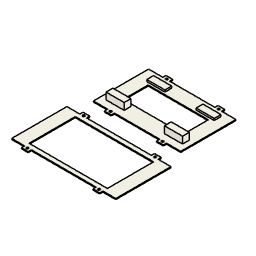
SD XL Bracket (Autodesk Fusion 360 design; units mm, degrees)
Autodesk Fusion 360 part; units mm, degrees
note: some values were not read from the file. Set by a fixed rule: which sketch regions a step uses.
sketch "Sketch1" plane through (0, 0, 0) normal (0, 0, 1) x (1, 0, 0) in component "SD XL Back"
  line L0 (0, 0) -> (0, 5) construction
  line L1 (-91.5, 117) -> (91.5, 117)
  line L2 (91.5, 117) -> (91.5, 5)
  line L3 (91.5, 5) -> (-91.5, 5)
  line L4 (-91.5, 5) -> (-91.5, 117)
  line L5 (-74.5, 111) -> (-34.5, 111)
  line L6 (-34.5, 111) -> (-34.5, 96)
  line L7 (-34.5, 96) -> (-74.5, 96)
  line L8 (-74.5, 96) -> (-74.5, 111)
  line L9 (34.5, 111) -> (74.5, 111)
  line L10 (74.5, 111) -> (74.5, 96)
  line L11 (74.5, 96) -> (34.5, 96)
  line L12 (34.5, 96) -> (34.5, 111)
  line L13 (-84.5, 31) -> (-44.5, 31)
  line L14 (-44.5, 31) -> (-44.5, 16)
  line L15 (-44.5, 16) -> (-84.5, 16)
  line L16 (-84.5, 16) -> (-84.5, 31)
  line L17 (44.5, 31) -> (84.5, 31)
  line L18 (84.5, 31) -> (84.5, 16)
  line L19 (84.5, 16) -> (44.5, 16)
  line L20 (44.5, 16) -> (44.5, 31)
  line L21 (-66.5, 91) -> (66.5, 91)
  line L22 (66.5, 91) -> (66.5, 36)
  line L23 (66.5, 36) -> (-66.5, 36)
  line L24 (-66.5, 36) -> (-66.5, 91)
  line L25 (0, 117) -> (0, 91) construction
  line L26 (0, 5) -> (0, 36) construction
  line L27 (-96.5, 0) -> (-96.5, 122)
  line L28 (96.5, 122) -> (96.5, 0)
  line L29 (-65, 117) -> (-50, 117)
  line L30 (-50, 117) -> (-50, 129)
  line L31 (-50, 129) -> (-65, 129)
  line L32 (-65, 129) -> (-65, 117)
  line L33 (50, 117) -> (65, 117)
  line L34 (65, 117) -> (65, 129)
  line L35 (65, 129) -> (50, 129)
  line L36 (50, 129) -> (50, 117)
  line L37 (57.5, 129) -> (57.5, 117) construction
  line L38 (-57.5, 129) -> (-57.5, 117) construction
  circle A0 centre (57.5, 123) radius 2.5
  circle A1 centre (-57.5, 123) radius 2.5
  line L39 (-96.5, 122) -> (-65, 122)
  line L40 (-50, 122) -> (50, 122)
  line L41 (65, 122) -> (96.5, 122)
  line L42 (-50, 5) -> (-65, 5)
  line L43 (-65, 5) -> (-65, -7)
  line L44 (-65, -7) -> (-50, -7)
  line L45 (-50, -7) -> (-50, 5)
  line L46 (50, 5) -> (65, 5)
  line L47 (65, 5) -> (65, -7)
  line L48 (65, -7) -> (50, -7)
  line L49 (50, -7) -> (50, 5)
  line L50 (-57.5, 5) -> (-57.5, -7) construction
  line L51 (57.5, 5) -> (57.5, -7) construction
  circle A2 centre (-57.5, -1) radius 2.5
  circle A3 centre (57.5, -1) radius 2.5
  line L52 (-65, 0) -> (-96.5, 0)
  line L53 (96.5, 0) -> (65, 0)
  line L54 (50, 0) -> (-50, 0)
  dimension "d1" = 5
  dimension "d2" = 183
  dimension "d5" = 112
  dimension "d8" = 40
  dimension "d9" = 15
  dimension "d10" = 17
  dimension "d11" = 17
  dimension "d12" = 7
  dimension "d13" = 7
  dimension "d14" = 11
  dimension "d15" = 11
  dimension "d19" = 25
  dimension "d28" = 12
  dimension "d29" = 15
  dimension "d31" = 50
  dimension "d32" = 50
  dimension "d33" = 5
  dimension "d41" = 6
  dimension "d42" = 5
  dimension "d43" = 5
  dimension "d44" = 26
  constraint coincident L0.start origin
  constraint vertical L0
  constraint horizontal L1
  constraint vertical L2
  constraint horizontal L3
  constraint vertical L4
  constraint midpoint L0.end L3
  constraint horizontal L5
  constraint vertical L6
  constraint horizontal L7
  constraint vertical L8
  constraint horizontal L9
  constraint vertical L10
  constraint horizontal L11
  constraint vertical L12
  constraint equal L7 L11
  constraint equal L6 L12
  constraint horizontal L13
  constraint vertical L14
  constraint horizontal L15
  constraint vertical L16
  constraint horizontal L17
  constraint vertical L18
  constraint horizontal L19
  constraint vertical L20
  constraint equal L7 L15
  constraint equal L7 L19
  constraint equal L6 L14
  constraint equal L6 L18
  constraint horizontal L21
  constraint vertical L22
  constraint horizontal L23
  constraint vertical L24
  constraint midpoint L1 L25.start
  constraint perpendicular L1 L25
  constraint midpoint L21 L25.end
  constraint perpendicular L3 L26
  constraint midpoint L23 L26.end
  constraint horizontal L29
  constraint vertical L30
  constraint horizontal L31
  constraint vertical L32
  constraint coincident L1 L29.start
  constraint horizontal L33
  constraint vertical L34
  constraint horizontal L35
  constraint vertical L36
  constraint coincident L1 L33.start
  constraint equal L30 L36
  constraint equal L31 L35
  constraint midpoint L35 L37.start
  constraint midpoint L33 L37.end
  constraint midpoint L31 L38.start
  constraint midpoint L29 L38.end
  constraint midpoint L37 A0.centre
  constraint midpoint L38 A1.centre
  constraint equal A0 A1
  constraint coincident L30 L40.start
  constraint collinear L39 L40
  constraint coincident L32 L39.end
  constraint coincident L36 L40.end
  constraint collinear L40 L41
  constraint coincident L34 L41.start
  constraint horizontal L42
  constraint vertical L43
  constraint horizontal L44
  constraint vertical L45
  constraint horizontal L46
  constraint vertical L47
  constraint horizontal L48
  constraint vertical L49
  constraint equal L32 L43
  constraint equal L32 L49
  constraint equal L31 L44
  constraint equal L31 L48
  constraint collinear L36 L49
  constraint collinear L30 L45
  constraint midpoint L42 L50.start
  constraint midpoint L44 L50.end
  constraint midpoint L46 L51.start
  constraint midpoint L48 L51.end
  constraint midpoint L50 A2.centre
  constraint midpoint L51 A3.centre
  constraint equal A1 A2
  constraint equal A1 A3
  constraint collinear L3 L42
  constraint collinear L3 L46
  constraint coincident L43 L52.start
  constraint collinear L52 L53
  constraint coincident L45 L54.end
  constraint coincident L49 L54.start
  constraint collinear L53 L54
  constraint coincident L47 L53.end
  constraint collinear L5 L9
  measures "d1" distance of L0.start L0.end
  measures "d2" distance of L1.start L1.end
  measures "d5" distance of L1.start L3.end
  measures "d8" distance of L6.end L7.end
  measures "d9" distance of L5.end L6.end
  measures "d10" distance of L4 L5.start
  measures "d11" distance of L2 L10
  measures "d12" distance of L4 L16
  measures "d13" distance of L2 L18
  measures "d14" distance of L3 L15
  measures "d15" distance of L3 L19
  measures "d19" distance of L2 L22
  measures "d28" distance of L29.start L31.end
  measures "d29" distance of L30.end L31.end
  measures "d31" distance of L25.start L29.end
  measures "d32" distance of L25.start L33.start
  measures "d33" diameter of A1
  measures "d41" distance of L1 L5
  measures "d42" distance of L13 L23
  measures "d43" distance of L7 L21
  measures "d44" distance of L1 L21
extrude "Extrude1" add sketch "Sketch1" against normal blind 2 contours L1 L3 L4 L27 L32 L39 L43 L52 | L1 L2 L3 L4 L29 L33 L42 L46 | L1 L29 L30 L31 L32 | L1 L30 L36 L40 | L3 L42 L43 L44 L45 | L1 L33 L34 L35 L36 | L3 L45 L49 L54 | L1 L2 L3 L28 L34 L41 L47 L53 | L3 L46 L47 L48 L49 | L5 L6 L7 L8 | L9 L10 L11 L12 | L13 L14 L15 L16 | L17 L18 L19 L20 makes body 1 in component "SD XL Back"
extrude "Extrude2" add sketch "Sketch1" along normal blind 4 contours L5 L6 L7 L8 | L9 L10 L11 L12 bodies 1 in component "SD XL Back"
extrude "Extrude3" add sketch "Sketch1" along normal blind 15 contours L13 L14 L15 L16 | L17 L18 L19 L20 bodies 1 in component "SD XL Back"
sketch "Sketch1 (2)" plane through (0, 0, 0) normal (0, 0, 1) x (1, 0, 0) in component "SD XL Front"
  line L0 (0, 0) -> (0, -50) construction
  line L1 (-86.5, -50) -> (86.5, -50)
  line L2 (86.5, -50) -> (86.5, -152)
  line L3 (86.5, -152) -> (-86.5, -152)
  line L4 (-86.5, -152) -> (-86.5, -50)
  line L5 (-115, -162) -> (-115, -40)
  line L6 (115, -40) -> (115, -162)
  line L7 (-86.5, -33) -> (-71.5, -33)
  line L8 (-71.5, -33) -> (-71.5, -45)
  line L9 (-71.5, -45) -> (-86.5, -45)
  line L10 (-86.5, -45) -> (-86.5, -33)
  line L11 (-50, 129) -> (-65, 129)
  line L12 (-65, 129) -> (-65, 117)
  line L13 (-79, -33) -> (-79, -45) construction
  circle A0 centre (-79, -39) radius 2.5
  circle A1 centre (-57.5, 123) radius 2.5 construction
  line L14 (-71.5, -40) -> (-71.5, -50) construction
  line L15 (71.5, -33) -> (86.5, -33)
  line L16 (86.5, -33) -> (86.5, -45)
  line L17 (86.5, -45) -> (71.5, -45)
  line L18 (71.5, -45) -> (71.5, -33)
  line L19 (79, -33) -> (79, -45) construction
  circle A2 centre (79, -39) radius 2.5
  line L20 (-71.5, -152) -> (-71.5, -162) construction
  line L21 (-86.5, -157) -> (-71.5, -157)
  line L22 (-71.5, -157) -> (-71.5, -169)
  line L23 (-71.5, -169) -> (-86.5, -169)
  line L24 (-86.5, -169) -> (-86.5, -157)
  line L25 (71.5, -157) -> (86.5, -157)
  line L26 (86.5, -157) -> (86.5, -169)
  line L27 (86.5, -169) -> (71.5, -169)
  line L28 (71.5, -169) -> (71.5, -157)
  line L29 (79, -157) -> (79, -169) construction
  line L30 (-79, -157) -> (-79, -169) construction
  circle A3 centre (79, -163) radius 2.5
  circle A4 centre (-79, -163) radius 2.5
  line L31 (-115, -40) -> (-86.5, -40)
  line L32 (-71.5, -40) -> (71.5, -40)
  line L33 (86.5, -40) -> (115, -40)
  line L34 (115, -162) -> (86.5, -162)
  line L35 (71.5, -162) -> (-71.5, -162)
  line L36 (-86.5, -162) -> (-115, -162)
  dimension "d34" = 50
  dimension "d35" = 173
  dimension "d37" = 102
  dimension "d45" = 230
  constraint coincident L0.start origin
  constraint vertical L0
  constraint horizontal L1
  constraint vertical L2
  constraint horizontal L3
  constraint vertical L4
  constraint midpoint L0.end L1
  constraint horizontal L7
  constraint vertical L8
  constraint horizontal L9
  constraint vertical L10
  constraint equal L7 L11
  constraint equal L8 L12
  constraint midpoint L7 L13.start
  constraint midpoint L9 L13.end
  constraint midpoint L13 A0.centre
  constraint equal A0 A1
  constraint coincident L14.start L31
  constraint coincident L1 L14.end
  constraint perpendicular L1 L14
  constraint midpoint L8.end L14
  constraint collinear L4 L10
  constraint horizontal L15
  constraint vertical L16
  constraint horizontal L17
  constraint vertical L18
  constraint equal L7 L15
  constraint equal L8 L18
  constraint midpoint L15 L19.start
  constraint midpoint L17 L19.end
  constraint midpoint L19 A2.centre
  constraint equal A0 A2
  constraint collinear L2 L16
  constraint collinear L7 L15
  constraint coincident L3 L20.start
  constraint coincident L20.end L34
  constraint perpendicular L20 L34
  constraint horizontal L21
  constraint vertical L22
  constraint horizontal L23
  constraint vertical L24
  constraint horizontal L25
  constraint vertical L26
  constraint horizontal L27
  constraint vertical L28
  constraint equal L10 L24
  constraint equal L10 L28
  constraint equal L9 L23
  constraint equal L17 L27
  constraint collinear L2 L26
  constraint collinear L4 L24
  constraint midpoint L20 L21.end
  constraint collinear L23 L27
  constraint midpoint L25 L29.start
  constraint midpoint L27 L29.end
  constraint midpoint L21 L30.start
  constraint midpoint L23 L30.end
  constraint midpoint L29 A3.centre
  constraint midpoint L30 A4.centre
  constraint equal A0 A4
  constraint equal A0 A3
  constraint coincident L10 L31.end
  constraint collinear L31 L32
  constraint coincident L18 L32.end
  constraint collinear L32 L33
  constraint coincident L16 L33.start
  constraint coincident L26 L34.end
  constraint collinear L34 L35
  constraint coincident L28 L35.start
  constraint collinear L35 L36
  constraint coincident L24 L36.start
  constraint equal L31 L33
  constraint vertical L6
  measures "d34" distance of L0.start L0.end
  measures "d35" distance of L1.start L1.end
  measures "d37" distance of L1.start L3.end
  measures "d45" distance of L5 L6
extrude "Extrude1'" add sketch "Sketch1 (2)" against normal blind 2 separate body makes body 2 in component "SD XL Front"
component "SD XL Back" placed x (1, 0, 0) y (0, 1, 0) z (0, 0, 1) at (0, 0, 0)
component "SD XL Front" placed x (1, 0, 0) y (0, 1, 0) z (0, 0, 1) at (0, 0, 0)
equation "d2 = SD_XL_Width"
equation "SD_XL_Width = 183 mm"
equation "SD_XL_Height = 112 mm"
equation "d5 = SD_XL_Height"
equation "SD_XL_Top_Depth = 34 mm"
equation "SD_XL_Bottom_Depth = 23 mm"
equation "d11 = d10"
equation "d13 = d12"
equation "d15 = d14"
equation "d16 = 25 mm"
equation "d19 = d16"
equation "Frame_Depth = 38 mm"
equation "d23 = Frame_Depth - SD_XL_Top_Depth"
equation "d25 = Frame_Depth - SD_XL_Bottom_Depth"
equation "d32 = d31"
equation "d35 = SD_XL_Width - 10 mm"
equation "d37 = SD_XL_Height - 10 mm"
equation "d43 = d42"
